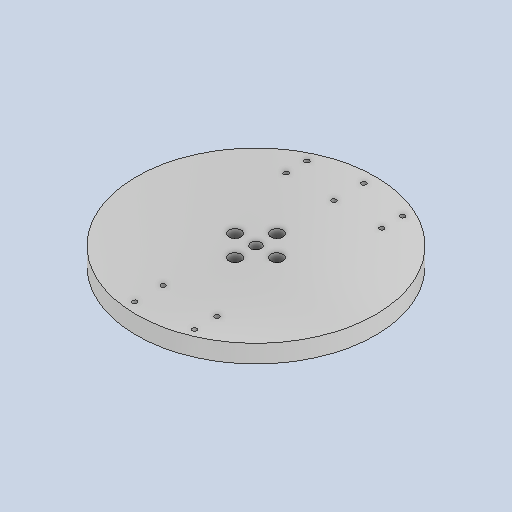
# Autodesk Inventor part: axis_2_bottom_frame
Saved by Autodesk Inventor 2024.1 (Build 281209000, 209)
## iProperties
Created: 2023-08-30
Part Number: axis_2_bottom_frame
Material: Aluminum 6061-AHC
Document SubType Name: Modeling
Designer: chanh
Density: 2.7 g/cm^3
Appearance: Aluminum - Dark
Author: chanh
Autodesk Inventor part; units mm, degrees
ref_plane "YZ Plane" through (0, 0, 0) normal (1, 0, 0) x (0, 1, 0)
ref_plane "XZ Plane" through (0, 0, 0) normal (0, 1, 0) x (-1, 0, 0)
ref_plane "XY Plane" through (0, 0, 0) normal (0, 0, 1) x (1, 0, 0)
sketch "Sketch1" plane through (0, 0, 0) normal (0, 1, 0) x (-1, 0, 0)
  circle A0 centre (0, 0) radius 40
  dimension "d0" = 80
  constraints: 1 centre point, 1 coincident
  measures "d0" diameter of A0
extrude "Extrusion1" add sketch "Sketch1" along normal blind 6
sketch "Sketch2" plane through (0, 0, 0) normal (0, -1, 0) x (1, 0, 0)
  circle A0 centre (0, 0) radius 35.15 projected
  circle A1 centre (0, 0) radius 24.85 projected
  point P0 (0, 0)
extrude "Extrusion2" cut sketch "Sketch2" against normal blind 1.43
sketch "Sketch3" plane through (0, 6, 0) normal (0, 1, 0) x (1, 0, 0)
  circle A0 centre (-7, 0) radius 0.7835 projected
  circle A1 centre (0, 7) radius 0.7835 projected
  circle A2 centre (0, -7) radius 0.7835 projected
  circle A3 centre (7, 0) radius 0.7835 projected
  point P0 (0, 0)
hole "Hole1" at (-7, 6, 0) at (0, 6, 7) at (7, 6, 0) at (0, 6, -7) direction (0, -1, 0) diameter 2.1 end through all
sketch "Sketch4" plane through (0, 6, 0) normal (0, 1, 0) x (1, 0, 0)
  circle A0 centre (0, 7) radius 1.05 projected
  circle A1 centre (7, 0) radius 1.05 projected
  circle A2 centre (0, -7) radius 1.05 projected
  circle A3 centre (-7, 0) radius 1.05 projected
  circle A4 centre (0, 0) radius 40 projected
  circle A5 centre (-7, 0) radius 2.05
  circle A6 centre (0, -7) radius 2.05
  circle A7 centre (7, 0) radius 2.05
  circle A8 centre (0, 7) radius 2.05
  dimension "d12" = 4.1
  constraints: 4 centre point, 4 coincident, 3 equal radius
  measures "d12" diameter of A5
extrude "Extrusion3" cut sketch "Sketch4" against normal blind 3 contours A5 | A6 | A7 | A8
sketch "Sketch5" plane through (0, 6, 0) normal (0, 1, 0) x (1, 0, 0)
  circle A0 centre (0, 0) radius 1.75 projected
extrude "Extrusion4" cut sketch "Sketch5" against normal through all
sketch "Sketch6" plane through (0, 0, 0) normal (0, -1, 0) x (1, 0, 0)
  circle A0 centre (0, 0) radius 2.75
  dimension "d17" = 5.5
  constraints: 1 centre point, 1 coincident
  measures "d17" diameter of A0
extrude "Extrusion5" cut sketch "Sketch6" against normal blind 1.5
sketch "Sketch7" plane through (0, 6, 0) normal (0, 1, 0) x (1, 0, 0)
  circle A0 centre (-4, -36.56) radius 1.05 projected
  circle A1 centre (-4, -27.06) radius 1.05 projected
  circle A2 centre (14, -27.06) radius 1.05 projected
  circle A3 centre (14, -34.56) radius 1.05 projected
  circle A4 centre (16, 26.06) radius 1.05 projected
  circle A5 centre (16, 33.06) radius 1.05 projected
  circle A6 centre (0, 36.06) radius 1.05 projected
  circle A7 centre (0, 26.06) radius 1.05 projected
  circle A8 centre (-16, 33.06) radius 1.05 projected
  circle A9 centre (-16, 26.06) radius 1.05 projected
  point P0 (0, 0)
hole "Hole2" at (-16, 6, -33.06) at (0, 6, -36.06) at (16, 6, -33.06) at (16, 6, -26.06) at (0, 6, -26.06) at (-16, 6, -26.06) at (-4, 6, 27.06) at (14, 6, 27.06) at (14, 6, 34.56) at (-4, 6, 36.56) direction (0, -1, 0) diameter 1.567 depth 3 thread size "M2x0.4" class "6H" standard "ISO Metric profile"
body "Solid1"
